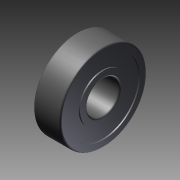
# Autodesk Inventor part: bearing_6201
Saved by Autodesk Inventor 2011 SP1 (Build 150282100, 282)
## iProperties
Created: 2016-03-21
Part Number: bearing_6201
Catalog Web Link: www.cadenas.de
Description: 6000_bearing-Deep Groove Ball Bearings
Vendor: MISUMI
Document SubType Name: Modeling
Designer: psAdmin
Manufacturer: MISUMI
Mass: 6.60755 g
Surface Area: 28.1366 cm^2
Volume: 6.60755 cm^3
Density: 1 g/cm^3
Category: PARTsolutions
Company: MISUMI
Title: bearing_6201
Author: Cadenas PARTsolutions
Comments: Deep Groove Ball Bearings
PSOL_IDENT_0: {$CADENAS_DATA\23d-libs\misumi\metric\accessories\bearing_6000.prj},173 {VTYP=3D},{NB=bearing_6201},
PSOL_IDENT_1: {LINA=bearing_6201},{NN=6000_bearing},{DATE=22.04.2015 10:37:55},{GEOMDATE=24.10.2013 00:00:00},{VER
PSOL_IDENT_2: SION=},{LINEID=100},{LINESUBID=-1},{WBVAR=}  {NB=bearing_6201},{LINA=bearing_6201},{KT=DUMMY},{PN=be
PSOL_IDENT_3: aring_6201},{BN=6201},{DD=12},{D=32},{B=10},{RR=0.6},{DSMIN=16.0},{DS1=17.00},{DSMAX=17.00},{DDHH=28
PSOL_IDENT_4: .0},{R=0.6},{R1=0.400},{R2=0.500},{MASS=37},{MASS11=37},{AA=9.1340},{BB=2.6000},{CC=2.7000},{DD1=30.
PSOL_IDENT_5: 150}
NN: 6000_bearing
NT: Deep Groove Ball Bearings
NB: bearing_6201
NBSYN: $PN.
LINA: bearing_6201
PN: bearing_6201
BN: 6201
DD: 12
D: 32
B: 10
RR: 0.6
DSMIN: 16.0
DDHH: 28.0
R: 0.6
MASS11: 37
SUPPLIER: MISUMI
ARTICLENO: bearing_6201
BOMINFO: bearing_6201
CREATOR: CADENAS GmbH
Autodesk Inventor part; units mm, degrees
sketch "Sketch_1" plane through (0, 0, 0) normal (0, 0, 1) x (1, 0, 0)
  line L0 (10, 0) -> (0, 0)
  line L1 (0, 15.4) -> (0, 13.4)
  line L2 (0, 13.4) -> (0.433, 13.4)
  line L3 (0.433, 13.4) -> (0.433, 8.7)
  line L4 (0.433, 8.7) -> (0, 8.7)
  line L5 (0, 8.7) -> (0, 6.6)
  arc A0 (0, 6.6) -> (0.6, 6) centre (0.6, 6.6) ccw
  line L6 (0.6, 6) -> (9.4, 6)
  arc A1 (9.4, 6) -> (10, 6.6) centre (9.4, 6.6) ccw
  line L7 (10, 6.6) -> (10, 8.7)
  line L8 (10, 8.7) -> (9.567, 8.7)
  line L9 (9.567, 8.7) -> (9.567, 13.4)
  line L10 (9.567, 13.4) -> (10, 13.4)
  line L11 (10, 13.4) -> (10, 15.4)
  arc A2 (10, 15.4) -> (9.4, 16) centre (9.4, 15.4) ccw
  line L12 (9.4, 16) -> (0.6, 16)
  arc A3 (0.6, 16) -> (0, 15.4) centre (0.6, 15.4) ccw
  constraints: 26 end point, 8 point on circle, 4 centre point
revolve "Revolution1" add sketch "Sketch_1" angle 360 about axis through (10, 0, 0) along (1, 0, 0)
ref_plane "center_point_XY" through (5, 0, 0) normal (1, 0, 0) x (0, 0, -1)
ref_plane "center_point_YZ" through (5, 0, 0) normal (0, 0, -1) x (0, 1, 0)
ref_plane "center_point_ZX" through (5, 0, 0) normal (0, 1, 0) x (1, 0, 0)
ref_plane "to_housing_XY" through (0, 0, 0) normal (1, 0, 0) x (0, 0, -1)
ref_plane "to_housing_YZ" through (0, 0, 0) normal (0, 0, -1) x (0, 1, 0)
ref_plane "to_housing_ZX" through (0, 0, 0) normal (0, 1, 0) x (1, 0, 0)
ref_plane "to_ring_XY" through (9.134, 0, 0) normal (1, 0, 0) x (0, 0, -1)
ref_plane "to_ring_YZ" through (9.134, 0, 0) normal (0, 0, -1) x (0, 1, 0)
ref_plane "to_ring_ZX" through (9.134, 0, 0) normal (0, 1, 0) x (1, 0, 0)
body "Solid1"
